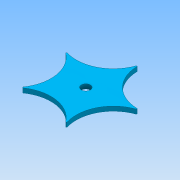
# Autodesk Inventor part: Pancake_Star
Saved by Autodesk Inventor 2018.1 (Build 221171000, 171)
## iProperties
Created: 2019-02-11
Part Number: Pancake_Star
Material: PC/ABS Plastic
Document SubType Name: Modeling
Designer: James
Density: 0.357273 g/cm^3
Appearance: Sky Blue Medium
Mass: 1.39714 g
Surface Area: 32.4947 cm^2
Volume: 3.91056 cm^3
Author: James
Autodesk Inventor part; units mm, degrees
ref_plane "YZ Plane" through (0, 0, 0) normal (1, 0, 0) x (0, 1, 0)
ref_plane "XZ Plane" through (0, 0, 0) normal (0, 1, 0) x (-1, 0, 0)
ref_plane "XY Plane" through (0, 0, 0) normal (0, 0, 1) x (1, 0, 0)
sketch "Sketch1" plane through (0, 0, 0) normal (0, 0, 1) x (1, 0, 0)
  circle A0 centre (0, 0) radius 30
  dimension "d0" = 60
  constraints: 1 centre point, 1 coincident
  measures "d0" diameter of A0
extrude "Extrusion1" add sketch "Sketch1" along normal blind 3
sketch "Sketch2" plane through (0, 0, 3) normal (0, 0, 1) x (1, 0, 0)
  circle A0 centre (0, 0) radius 30 projected
  circle A1 centre (30, 30) radius 25
  dimension "d6" = 50
  dimension "d7" = 30
  dimension "d8" = 30
  constraints: 1 centre point
  measures "d6" diameter of A1
  measures "d7" horizontal distance of point (0, 0) A1.centre
  measures "d8" horizontal distance of A1.centre point (0, 0)
extrude "Extrusion2" cut sketch "Sketch2" against normal through all contours A1 A0 | A0 A1 picked at (18.8229, 17.5315) picked at (30.2504, 29.5845)
pattern_circular "Circular Pattern1" count 5 over 360 about axis through (0, 0, -10) along (0, 0, 1) of "Extrusion2"
sketch "Sketch3" plane through (0, 0, 3) normal (0, 0, 1) x (1, 0, 0)
  point P0 (0, 0)
  point P1 (0, 0)
  constraints: 1 coincident
hole "Hole1" at (0, 0, 3) direction (0, 0, -1) diameter 6 end through all
equation "\"d8\" = d7"
body "Solid1"
